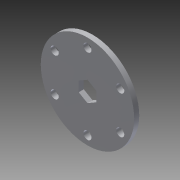
# Autodesk Inventor part: wheelhubthing
Saved by Autodesk Inventor 2014 SP1 (Build 180222100, 222)
## iProperties
Created: 2014-01-06
Part Number: wheelhubthing
Material: Aluminum 6061
Document SubType Name: Modeling
Designer: Arpan
Density: 2.71 g/cm^3
Appearance: Aluminum - Flat
Mass: 21.3672 g
Surface Area: 59.7753 cm^2
Volume: 7.88456 cm^3
Author: Arpan
Autodesk Inventor part; units mm, degrees
note: some values were not read from the file. Chosen so that the rebuilt part matches the saved one: sketch regions of "Extrusion1".
ref_plane "YZ Plane" through (0, 0, 0) normal (1, 0, 0) x (0, 1, 0)
ref_plane "XZ Plane" through (0, 0, 0) normal (0, 1, 0) x (-1, 0, 0)
ref_plane "XY Plane" through (0, 0, 0) normal (0, 0, 1) x (1, 0, 0)
sketch "Sketch1" plane through (0, 0, 0) normal (0, 0, 1) x (1, 0, 0)
  arc A0 (24.3719, -16.0061) -> (18.9457, -6.6082) centre (20.6227, -11.9054) ccw
  arc A1 (18.9457, -6.6082) -> (15.375, -3.3543) centre (0, -23.8125) ccw
  arc A2 (15.4859, -6.1082) -> (15.375, -3.3543) centre (14.3062, -4.7765) ccw
  arc A3 (15.4859, -6.1082) -> (13.3187, -9.3259) centre (20.6222, -11.9062) ccw
  arc A4 (10.5541, -10.1415) -> (13.3187, -9.3259) centre (11.6413, -8.7333) ccw
  arc A5 (10.5541, -10.1415) -> (6.5626, -7.8369) centre (0, -23.8125) ccw
  arc A6 (5.8865, -5.0351) -> (6.5626, -7.8369) centre (7.2386, -6.1913) ccw
  arc A7 (5.8865, -5.0351) -> (7.5891, -1.5492) centre (-0.0005, -0.0009) ccw
  arc A8 (10.0295, -0.2681) -> (7.5891, -1.5492) centre (9.3323, -1.9049) ccw
  arc A9 (10.0295, -0.2681) -> (5.4257, 1.1973) centre (0, -23.8125) ccw
  arc A10 (5.4257, 1.1973) -> (-5.4257, 1.1973) centre (0, 0) ccw
  arc A11 (-5.4257, 1.1973) -> (-10.0298, -0.2683) centre (0, -23.8125) ccw
  arc A12 (-7.5894, -1.5492) -> (-10.0298, -0.2683) centre (-9.3326, -1.905) ccw
  arc A13 (-7.5894, -1.5492) -> (-5.8864, -5.0349) centre (0, 0) ccw
  arc A14 (-6.5624, -7.8369) -> (-5.8864, -5.0349) centre (-7.2384, -6.1912) ccw
  arc A15 (-6.5624, -7.8369) -> (-10.554, -10.1414) centre (0, -23.8125) ccw
  arc A16 (-13.3185, -9.326) -> (-10.554, -10.1414) centre (-11.6411, -8.7331) ccw
  arc A17 (-13.3185, -9.326) -> (-15.486, -6.1085) centre (-20.6217, -11.9071) ccw
  arc A18 (-15.3753, -3.3545) -> (-15.486, -6.1085) centre (-14.3064, -4.7767) ccw
  arc A19 (-15.3753, -3.3545) -> (-18.9467, -6.6093) centre (0, -23.8125) ccw
  arc A20 (-18.9467, -6.6093) -> (-24.3721, -16.0067) centre (-20.6217, -11.9071) ccw
  arc A21 (-24.3721, -16.0067) -> (-25.4048, -20.7264) centre (0, -23.8125) ccw
  arc A22 (-23.0753, -19.2535) -> (-25.4048, -20.7264) centre (-23.6387, -20.941) ccw
  arc A23 (-23.0753, -19.2535) -> (-19.2051, -19.5215) centre (-20.6222, -11.9063) ccw
  arc A24 (-17.1165, -21.5079) -> (-19.2051, -19.5215) centre (-18.8796, -21.2705) ccw
  arc A25 (-17.1165, -21.5079) -> (-17.1165, -26.1169) centre (0, -23.8125) ccw
  arc A26 (-19.2049, -28.1034) -> (-17.1165, -26.1169) centre (-18.8797, -26.3543) ccw
  arc A27 (-19.2049, -28.1034) -> (-23.0751, -28.3718) centre (-20.6212, -35.7187) ccw
  arc A28 (-25.4048, -26.8989) -> (-23.0751, -28.3718) centre (-23.6387, -26.6843) ccw
  arc A29 (-25.4048, -26.8989) -> (-24.3714, -31.6203) centre (0, -23.8125) ccw
  arc A30 (-24.3714, -31.6203) -> (-18.9453, -41.0172) centre (-20.6207, -35.7196) ccw
  arc A31 (-18.9453, -41.0172) -> (-15.375, -44.2707) centre (0, -23.8125) ccw
  arc A32 (-15.4859, -41.5168) -> (-15.375, -44.2707) centre (-14.3062, -42.8485) ccw
  arc A33 (-15.4859, -41.5168) -> (-13.3187, -38.2991) centre (-20.6222, -35.7188) ccw
  arc A34 (-10.5541, -37.4835) -> (-13.3187, -38.2991) centre (-11.6413, -38.8917) ccw
  arc A35 (-10.5541, -37.4835) -> (-6.5626, -39.7881) centre (0, -23.8125) ccw
  arc A36 (-5.8865, -42.5899) -> (-6.5626, -39.7881) centre (-7.2386, -41.4337) ccw
  arc A37 (-5.8865, -42.5899) -> (-7.5891, -46.0758) centre (0.0005, -47.6241) ccw
  arc A38 (-10.0295, -47.3569) -> (-7.5891, -46.0758) centre (-9.3323, -45.7201) ccw
  arc A39 (-10.0295, -47.3569) -> (-5.4236, -48.8227) centre (0, -23.8125) ccw
  arc A40 (-5.4236, -48.8227) -> (5.4278, -48.8218) centre (0.002, -47.625) ccw
  arc A41 (5.4278, -48.8218) -> (10.0298, -47.3567) centre (0, -23.8125) ccw
  arc A42 (7.5894, -46.0758) -> (10.0298, -47.3567) centre (9.3326, -45.72) ccw
  arc A43 (7.5894, -46.0758) -> (5.8864, -42.5901) centre (0, -47.625) ccw
  arc A44 (6.5624, -39.7881) -> (5.8864, -42.5901) centre (7.2384, -41.4338) ccw
  arc A45 (6.5624, -39.7881) -> (10.554, -37.4836) centre (0, -23.8125) ccw
  arc A46 (13.3185, -38.299) -> (10.554, -37.4836) centre (11.6411, -38.8919) ccw
  arc A47 (13.3185, -38.299) -> (15.486, -41.5165) centre (20.6217, -35.7179) ccw
  arc A48 (15.3753, -44.2705) -> (15.486, -41.5165) centre (14.3064, -42.8483) ccw
  arc A49 (15.3753, -44.2705) -> (18.9472, -41.0152) centre (0, -23.8125) ccw
  arc A50 (18.9472, -41.0152) -> (24.3725, -31.6169) centre (20.6237, -35.7179) ccw
  arc A51 (24.3725, -31.6169) -> (25.4048, -26.8986) centre (0, -23.8125) ccw
  arc A52 (23.0753, -28.3715) -> (25.4048, -26.8986) centre (23.6387, -26.684) ccw
  arc A53 (23.0753, -28.3715) -> (19.2051, -28.1035) centre (20.6222, -35.7187) ccw
  arc A54 (17.1165, -26.1171) -> (19.2051, -28.1035) centre (18.8796, -26.3545) ccw
  arc A55 (17.1165, -26.1171) -> (17.1165, -21.5081) centre (0, -23.8125) ccw
  arc A56 (19.2049, -19.5216) -> (17.1165, -21.5081) centre (18.8797, -21.2707) ccw
  arc A57 (19.2049, -19.5216) -> (23.0751, -19.2532) centre (20.6212, -11.9063) ccw
  arc A58 (25.4048, -20.7261) -> (23.0751, -19.2532) centre (23.6387, -20.9407) ccw
  arc A59 (25.4048, -20.7261) -> (24.3719, -16.0061) centre (0, -23.8125) ccw
  circle A60 centre (20.6227, -11.9054) radius 2.54
  circle A61 centre (20.6237, -35.7179) radius 2.54
  circle A62 centre (0.002, -47.625) radius 2.54
  circle A63 centre (-20.6207, -35.7196) radius 2.54
  circle A64 centre (-20.6217, -11.9071) radius 2.54
  circle A65 centre (0, 0) radius 2.54
  circle A66 centre (0, -23.8125) radius 14.2875
  circle A67 centre (0, -23.8125) radius 29.3688
  circle A68 centre (0, -23.8125) radius 6.35
  line L0 (0, 0) -> (0, -17.4625)
  line L1 (20.6227, -11.9054) -> (5.4278, -20.5169)
  line L2 (0, -17.4625) -> (5.4993, -20.6375)
  line L3 (5.4993, -20.6375) -> (5.4993, -26.9875)
  line L4 (5.4993, -26.9875) -> (0, -30.1625)
  line L5 (0, -30.1625) -> (-5.4993, -26.9875)
  line L6 (-5.4993, -26.9875) -> (-5.4993, -20.6375)
  line L7 (-5.4993, -20.6375) -> (0, -17.4625)
  dimension "d0" = 12.7
  constraints: 122 point on circle, 69 centre point, 16 end point, 3 coincident, 1 vertical, 13 other
  measures "d0" diameter of A68
extrude "Extrusion1" add sketch "Sketch1" along normal blind 3.175 contours A59 A58 A57 A56 A55 A54 A53 A52 A51 A50 A49 A48 A47 A46 A45 A44 A43 A42 A41 A40 A39 A38 A37 A36 A35 A34 A33 A32 A31 A30 A29 A28 A27 A26 A25 A24 A23 A22 A21 A20 A19 A18 A17 A16 A15 A14 A13 A12 A11 A10 A9 A8 A7 A6 A5 A4 A3 A2 A1 A0 | A0 A67 A50 A51 A52 A53 A54 A55 A56 A57 A58 A59 | A0 A1 A2 A3 A4 A5 A6 A7 A8 A9 A10 A67 | A10 A11 A12 A13 A14 A15 A16 A17 A18 A19 A20 A67 | A67 A40 A41 A42 A43 A44 A45 A46 A47 A48 A49 A50 | A20 A21 A22 A23 A24 A25 A26 A27 A28 A29 A30 A67 | A67 A30 A31 A32 A33 A34 A35 A36 A37 A38 A39 A40 | A66 L0 A68 L1 | L1 A68 L0 A66 | A68 L2 | L7 A68 | A68 L3 | L6 A68 | A68 L4 | L5 A68
body "Solid1"
